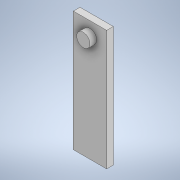
# Autodesk Inventor part: 수직축
Saved by Autodesk Inventor 2022 (Build 260153000, 153)
## iProperties
Created: 2022-10-28
Part Number: 수직축
Material: 일반
Document SubType Name: Modeling
Designer: whdls
Density: 1 g/cm^3
Appearance: 기본값
Author: whdls
Autodesk Inventor part; units mm, degrees
ref_plane "YZ Plane" through (0, 0, 0) normal (1, 0, 0) x (0, 1, 0)
ref_plane "XZ Plane" through (0, 0, 0) normal (0, 1, 0) x (-1, 0, 0)
ref_plane "XY Plane" through (0, 0, 0) normal (0, 0, 1) x (1, 0, 0)
sketch "스케치1" plane through (0, 0, 0) normal (0, 0, 1) x (1, 0, 0)
  line L0 (-2.5, -9) -> (2.5, -9)
  line L1 (2.5, -9) -> (2.5, 9)
  line L2 (2.5, 9) -> (-2.5, 9)
  line L3 (-2.5, 9) -> (-2.5, -9)
  line L4 (-2.5, -9) -> (2.5, 9) construction
  line L5 (2.5, -9) -> (-2.5, 9) construction
  point P0 (0, 0)
  dimension "d0" = 5
  dimension "d1" = 18
  constraints: 12 end point, 2 midpoint, 2 parallel, 1 horizontal, 1 perpendicular
  measures "d0" distance of L1.end L2.end
  measures "d1" distance of L0.end L1.end
extrude "돌출1" add sketch "스케치1" along normal blind 1
sketch "스케치2" plane through (0, 0, 1) normal (0, 0, 1) x (1, 0, 0)
  circle A0 centre (0, 7) radius 1
  line L0 (-3.5, 0) -> (3.5, 0) construction
  line L1 (0, -12.6) -> (0, 12.6) construction
  point P0 (0, 0)
  dimension "d4" = 2
  dimension "d5" = 7
  constraints: 1 centre point, 1 point on line
  measures "d4" diameter of A0
  measures "d5" distance of point (0, 0) A0.centre
extrude "돌출2" add sketch "스케치2" along normal blind 1
